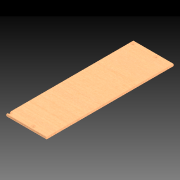
# Autodesk Inventor part: KB33-046-004-002 - Передняя пластина
Saved by Autodesk Inventor 2020 (Build 240168000, 168)
## iProperties
Created: 2021-06-25
Part Number: KB33-046-004-002 - Передняя пластина
Material: Дерево (вишня)
Document SubType Name: Modeling
Designer: Петров Иван
Mass: 54.8498 g
Surface Area: 464.898 cm^2
Volume: 87.0632 cm^3
Density: 0.63 g/cm^3
Appearance: Вишневое дерево — натуральный — со слабым глянцем
Author: Петров Иван
Autodesk Inventor part; units mm, degrees
ref_plane "YZ Plane" through (0, 0, 0) normal (1, 0, 0) x (0, 1, 0)
ref_plane "XZ Plane" through (0, 0, 0) normal (0, 1, 0) x (-1, 0, 0)
ref_plane "XY Plane" through (0, 0, 0) normal (0, 0, 1) x (1, 0, 0)
sketch "Эскиз1" plane through (0, 0, 0) normal (0, 1, 0) x (-1, 0, 0)
  line L0 (-2.6795, -79) -> (80.3545, -79)
  line L1 (-2.6795, 184) -> (80.3545, 184)
  circle A0 centre (30.7479, 178.5) radius 1.85
  circle A1 centre (78.7479, 178.5) radius 1.85
  circle A2 centre (76.0773, -73.5) radius 1.85
  circle A3 centre (28.0773, -73.5) radius 1.85
  line L2 (80.3545, 184) -> (-2.6795, 184)
  line L3 (-2.6795, 184) -> (-2.6795, -79)
  line L4 (-2.6795, -79) -> (80.3545, -79)
  line L5 (80.3545, -79) -> (80.3545, 184)
  point P0 (0, 0)
  point P1 (83.0251, -19)
  dimension "d7" = 5.5
  dimension "d8" = 48
  dimension "d9" = 4.2772
  dimension "d10" = 5.5
  dimension "d11" = 263
  dimension "d12" = 83.034
  constraints: 12 end point, 4 centre point, 2 horizontal, 2 parallel, 1 perpendicular
  measures "d7" distance from line of L0 A3.centre
  measures "d8" distance of A2.centre A3.centre
  measures "d9" distance from line of A2.centre L5
  measures "d10" distance from line of L0 A2.centre
  measures "d11" distance of L2.end L0.start
  measures "d12" distance of L0.start L0.end
extrude "Выдавливание1" add sketch "Эскиз1" along normal blind 4 contours L3 L1 L5 A1 L0
chamfer "Фаска1" distance 2 angle 45 4 edges at (-76.8979, 4, 178.5) (-28.8979, 4, 178.5) (-26.2273, 4, -73.5) (-74.2273, 4, -73.5)
